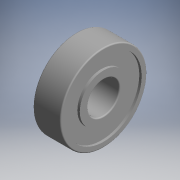
# Autodesk Inventor part: bearing_608
Saved by Autodesk Inventor 2017.3 (Build 213256000, 256)
## iProperties
Part Number: bearing_608
Material: Generic
Catalog Web Link: www.cadenas.de
Description: 600_bearing-Small Ball Bearings
Vendor: MISUMI
Document SubType Name: Modeling
Designer: partserver
Manufacturer: MISUMI
Mass: 2.09464 g
Surface Area: 14.1395 cm^2
Volume: 2.09464 cm^3
Density: 1 g/cm^3
Appearance: PSOLRGB-192-192-192
Category: PARTsolutions
Company: MISUMI
Title: bearing_608
Author: Cadenas PARTsolutions
Comments: Small Ball Bearings
PSOL_IDENT_0: {$CADENAS_DATA\23d-libs\misumi\metric\accessories\bearing_600.prj},168 {VTYP=3D},{NB=bearing_608},{L
PSOL_IDENT_1: INA=bearing_608},{NN=600_bearing},{DATE=17.06.2016 05:56:49},{GEOMDATE=24.10.2013 00:00:00},{VERSION=
PSOL_IDENT_2: },{LINEID=170},{WBVAR=},{WBNUMERIC=}  {NB=bearing_608},{LINA=bearing_608},{KT=DUMMY},{PN=bearing_608
PSOL_IDENT_3: },{BN=608},{DD=8.0},{D=22},{B=7.0},{RR=0.30},{DS=10.00},{DDHH=20.00},{R=0.30},{MASS=12},{A=5.8000},{
PSOL_IDENT_4: C=2.100},{BB=1.350}
NB: bearing_608
NN: 600_bearing
NT: Small Ball Bearings
NBSYN: $PN.
LINA: bearing_608
CATALOG: Misumi
PN: bearing_608
BN: 608
DD: 8
D: 22
B: 7
RR: 0.3
DS: 10
DDHH: 20
R: 0.3
MASS: 12
SUPPLIER: MISUMI
ARTICLENO: bearing_608
BOMINFO: bearing_608
CREATOR: CADENAS GmbH
Autodesk Inventor part; units mm, degrees
sketch "Sketch_1" plane through (0, 0, 0) normal (0, 0, 1) x (1, 0, 0)
  line L0 (6.7, 0) -> (0.3, 0)
  arc A0 (0, 4.3) -> (0.3, 4) centre (0.3, 4.3) ccw
  line L1 (0.3, 4) -> (6.7, 4)
  arc A1 (6.7, 4) -> (7, 4.3) centre (6.7, 4.3) ccw
  line L2 (7, 4.3) -> (7, 6.1)
  line L3 (7, 6.1) -> (6.4, 6.1)
  line L4 (6.4, 6.1) -> (6.4, 9.65)
  line L5 (6.4, 9.65) -> (7, 9.65)
  line L6 (7, 9.65) -> (7, 10.7)
  arc A2 (7, 10.7) -> (6.7, 11) centre (6.7, 10.7) ccw
  line L7 (6.7, 11) -> (0.3, 11)
  arc A3 (0.3, 11) -> (0, 10.7) centre (0.3, 10.7) ccw
  line L8 (0, 10.7) -> (0, 9.65)
  line L9 (0, 9.65) -> (0.6, 9.65)
  line L10 (0.6, 9.65) -> (0.6, 6.1)
  line L11 (0.6, 6.1) -> (0, 6.1)
  line L12 (0, 6.1) -> (0, 4.3)
  constraints: 26 end point, 8 point on circle, 4 centre point
revolve "Revolution1" add sketch "Sketch_1" angle 360 about axis through (6.7, 0, 0) along (1, 0, 0)
ref_plane "to_housing_XY" through (0, 0, 0) normal (1, 0, 0) x (0, 0, -1)
ref_plane "to_housing_YZ" through (0, 0, 0) normal (0, 0, -1) x (0, 1, 0)
ref_plane "to_housing_ZX" through (0, 0, 0) normal (0, 1, 0) x (1, 0, 0)
ref_plane "to_housing_center_XY" through (3.5, 0, 0) normal (1, 0, 0) x (0, 0, -1)
ref_plane "to_housing_center_YZ" through (3.5, 0, 0) normal (0, 0, -1) x (0, 1, 0)
ref_plane "to_housing_center_ZX" through (3.5, 0, 0) normal (0, 1, 0) x (1, 0, 0)
body "Solid1"
